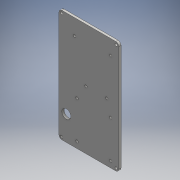
# Autodesk Inventor part: plate
Saved by Autodesk Inventor 2016 (Build 200138000, 138)
## iProperties
Created: 2018-07-05
Part Number: plate
Material: Generic
Document SubType Name: Modeling
Designer: andrew
Density: 1 g/cm^3
Appearance: Default
Author: andrew
Autodesk Inventor part; units mm, degrees
ref_plane "YZ Plane" through (0, 0, 0) normal (1, 0, 0) x (0, 1, 0)
ref_plane "XZ Plane" through (0, 0, 0) normal (0, 1, 0) x (-1, 0, 0)
ref_plane "XY Plane" through (0, 0, 0) normal (0, 0, 1) x (1, 0, 0)
sketch "Sketch1" plane through (0, 0, 0) normal (0, 1, 0) x (-1, 0, 0)
  line L0 (-40, 75) -> (40, 75)
  line L1 (40, 75) -> (40, -75)
  line L2 (40, -75) -> (-40, -75)
  line L3 (-40, -75) -> (-40, 75)
  line L4 (-40, 75) -> (40, -75) construction
  line L5 (40, 75) -> (-40, -75) construction
  point P0 (0, 0)
  dimension "d0" = 80
  dimension "d1" = 150
  constraints: 12 end point, 2 midpoint, 2 parallel, 1 horizontal, 1 perpendicular
  measures "d0" distance of L1.end L2.end
  measures "d1" distance of L0.end L1.end
extrude "Extrusion1" add sketch "Sketch1" along normal blind 3
sketch "Sketch2" plane through (0, 3, 0) normal (0, 1, 0) x (1, 0, 0)
  line L0 (-40, -75) -> (40, -75) construction
  line L1 (0, -75) -> (0, 75) construction
  line L2 (40, 75) -> (-40, 75) construction
  line L3 (40, -75) -> (40, 75) construction
  line L4 (40, 0) -> (-40, 0) construction
  line L5 (-40, 75) -> (-40, -75) construction
  line L6 (0, -75) -> (40, -75) construction
  line L7 (40, -75) -> (5, -75) construction
  line L8 (5, -75) -> (5, -35) construction
  line L9 (31.65, -69.3) -> (-21.65, -69.3) construction
  line L10 (-21.65, -69.3) -> (-21.65, -0.7) construction
  line L11 (-21.65, -0.7) -> (31.65, -0.7) construction
  line L12 (31.65, -0.7) -> (31.65, -69.3) construction
  line L13 (31.65, -69.3) -> (-21.65, -0.7) construction
  line L14 (-21.65, -69.3) -> (31.65, -0.7) construction
  line L15 (5, -69.3) -> (5, -55.3) construction
  line L16 (5, -55.3) -> (-21.65, -55.3) construction
  line L17 (5, -55.3) -> (31.65, -55.3) construction
  line L18 (-21.65, -54) -> (5, -54) construction
  line L19 (5, -54) -> (31.65, -54) construction
  line L20 (-21.65, -3.2) -> (5, -3.2) construction
  line L21 (5, -3.2) -> (31.65, -3.2) construction
  line L22 (31.65, -35) -> (29.15, -35) construction
  line L23 (29.15, -35) -> (29.15, -0.7) construction
  line L24 (29.15, -35) -> (29.15, -69.3) construction
  line L25 (24.05, -0.7) -> (24.05, -35) construction
  line L26 (24.05, -35) -> (24.05, -69.3) construction
  line L27 (-3.85, -0.7) -> (-3.85, -35) construction
  line L28 (-3.85, -35) -> (-3.85, -69.3) construction
  line L29 (-19.05, -0.7) -> (-19.05, -35) construction
  line L30 (-19.05, -35) -> (-19.05, -69.3) construction
  point P0 (0, 0)
  point P1 (-19.05, -54)
  point P2 (29.15, -55.3)
  point P3 (24.05, -3.2)
  point P4 (-3.85, -3.2)
  dimension "d4" = 35
  dimension "d5" = 40
  dimension "d6" = 53.3
  dimension "d7" = 68.6
  dimension "d8" = 14
  dimension "d9" = 1.3
  dimension "d10" = 50.8
  dimension "d11" = 2.5
  dimension "d12" = 5.1
  dimension "d13" = 27.9
  dimension "d14" = 15.2
  constraints: 54 end point, 15 point on line, 8 midpoint, 4 perpendicular, 3 horizontal, 2 parallel, 1 collinear, 5 other
  measures "d4" distance of L0.end L7.end
  measures "d5" distance of L7.end L8.end
  measures "d6" distance of L10.end L11.end
  measures "d7" distance of L9.end L10.end
  measures "d8" distance of L15.start L15.end
  measures "d9" distance between parallel lines of L16 L18
  measures "d10" distance between parallel lines of L18 L20
  measures "d11" distance of L22.start L22.end
  measures "d12" distance between parallel lines of L23 L25
  measures "d13" distance between parallel lines of L25 L27
  measures "d14" distance between parallel lines of L27 L29
hole "Hole1" at (-19.05, 3, 54) at (29.15, 3, 55.3) at (24.05, 3, 3.2) at (-3.85, 3, 3.2) direction (0, -1, 0) diameter 3.2 end through all
sketch "Sketch3" plane through (0, 3, 0) normal (0, 1, 0) x (1, 0, 0)
  line L0 (40, 75) -> (40, -75) construction
  line L1 (40, 75) -> (6.65, 75) construction
  line L2 (-40, 75) -> (40, 75) construction
  line L3 (6.65, 75) -> (6.65, 55) construction
  line L4 (-15.85, 16.5614) -> (29.15, 16.5614) construction
  line L5 (29.15, 16.5614) -> (29.15, 66.5614) construction
  line L6 (29.15, 66.5614) -> (-15.85, 66.5614) construction
  line L7 (-15.85, 66.5614) -> (-15.85, 16.5614) construction
  line L8 (-15.85, 16.5614) -> (29.15, 66.5614) construction
  line L9 (29.15, 16.5614) -> (-15.85, 66.5614) construction
  circle A0 centre (29.15, -55.3) radius 1.6 construction
  line L10 (29.15, -55.3) -> (40, -55.3) construction
  line L11 (29.15, -55.3) -> (29.15, 104.0464) construction
  point P0 (0, 0)
  point P1 (6.65, 41.5614)
  dimension "d22" = 33.35
  dimension "d23" = 20
  dimension "d24" = 45
  dimension "d25" = 50
  dimension "d26" = 10.85
  dimension "d27" = 10.85
  constraints: 20 end point, 3 point on line, 2 horizontal, 2 midpoint, 2 parallel, 2 vertical, 1 perpendicular
  measures "d22" distance of L0.start L1.end
  measures "d23" distance of L1.end L3.end
  measures "d24" distance of L6.end L5.end
  measures "d25" distance of L5.end L4.end
  measures "d26" distance of L10.start L10.end
  measures "d27" distance between parallel lines of L0 L5
hole "Hole2" at (-15.85, 3, -16.5614) at (-15.85, 3, -66.5614) at (29.15, 3, -16.5614) at (29.15, 3, -66.5614) direction (0, -1, 0) diameter 3.3 end through all
fillet "Fillet1" radius 4 4 edges at (40, 1.5, 75) (-40, 1.5, 75) (40, 1.5, -75) (-40, 1.5, -75)
sketch "Sketch4" plane through (0, 3, 0) normal (0, 1, 0) x (1, 0, 0)
  line L0 (-40, -75) -> (40, -75) projected
  line L1 (-40, 75) -> (-40, -75) projected
  line L2 (40, 75) -> (-40, 75) projected
  line L3 (40, -75) -> (40, 75) projected
  line L4 (36.5, 71.5) -> (-36.5, 71.5) construction
  line L5 (-36.5, 71.5) -> (-36.5, -71.5) construction
  line L6 (-36.5, -71.5) -> (36.5, -71.5) construction
  line L7 (36.5, -71.5) -> (36.5, 71.5) construction
  point P0 (0, 0)
  dimension "d36" = 3.5
  constraints: 8 end point, 4 coincident, 3 other
  measures "d36" distance between parallel lines of L3 L7
hole "Hole3" at (-36.5, 3, 71.5) at (36.5, 3, 71.5) at (36.5, 3, -71.5) at (-36.5, 3, -71.5) direction (0, -1, 0) diameter 3.3 end through all
hole "Hole4" at (-30.1058, 3, -41.9761) direction (0, -1, 0) diameter 12 end through all
body "Solid1"
